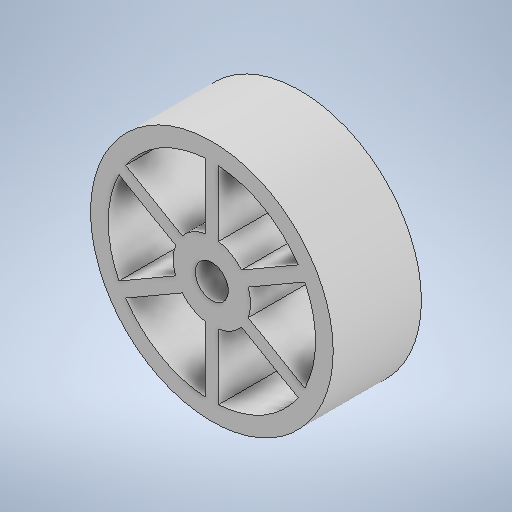
# Autodesk Inventor part: Wheel-D22A
Saved by Autodesk Inventor 2025.3 (Build 293356030, 356C)
## iProperties
Created: 2025-08-17
Part Number: Wheel-D22A
Material: 一般
Document SubType Name: Modeling
Designer: daisuke
Density: 1 g/cm^3
Appearance: 既定
Author: daisuke
Autodesk Inventor part; units mm, degrees
ref_plane "YZ Plane" through (0, 0, 0) normal (1, 0, 0) x (0, 1, 0)
ref_plane "XZ Plane" through (0, 0, 0) normal (0, 1, 0) x (-1, 0, 0)
ref_plane "XY Plane" through (0, 0, 0) normal (0, 0, 1) x (1, 0, 0)
sketch "スケッチ1" plane through (0, 0, 0) normal (0, 0, 1) x (1, 0, 0)
  circle A0 centre (0, 0) radius 3.5
  circle A1 centre (0, 0) radius 11
  circle A2 centre (0, 0) radius 9.4
  circle A3 centre (0, 0) radius 1.5
  dimension "HUB_DIA" = 7
  dimension "DIA" = 22
  dimension "d5" = 1.6
  dimension "d16" = 3
  constraints: 5 coincident, 4 centre point
  measures "HUB_DIA" diameter of A0
  measures "DIA" diameter of A1
  measures "d5" radial gap between concentric circles of A1 A2
  measures "d16" diameter of A3
extrude "ハブ＆リム" add sketch "スケッチ1" along normal blind 8
sketch "スケッチ2" plane through (0, 0, 0) normal (0, 0, 1) x (1, 0, 0)
  line L0 (-0.6, 2.5) -> (0.6, 2.5)
  line L1 (0.6, 2.5) -> (0.6, 10)
  line L2 (0.6, 10) -> (-0.6, 10)
  line L3 (-0.6, 10) -> (-0.6, 2.5)
  line L4 (0, 0) -> (0, 15.4673) construction
  point P0 (0, 2.5)
  dimension "d8" = 2.5
  dimension "d9" = 10
  dimension "d10" = 1.2
  constraints: 10 end point, 2 parallel, 1 horizontal, 1 midpoint, 1 perpendicular, 1 point on line, 1 vertical
  measures "d8" distance from line of L4.start L0
  measures "d9" distance from line of L4.start L2
  measures "d10" distance of L1.end L2.end
extrude "スポーク" add sketch "スケッチ2" along normal blind 8
pattern_circular "円形状パターン1" count 6 over 360 about axis through (0, 0, -10) along (0, 0, 1) of "スポーク"
